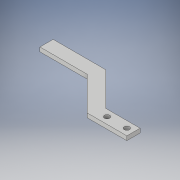
# Autodesk Inventor part: Pinza_dedo
Saved by Autodesk Inventor 2019 (Build 230136000, 136)
## iProperties
Created: 2020-02-07
Part Number: Pinza_dedo
Material: Generic
Document SubType Name: Modeling
Designer: Omar
Density: 1 g/cm^3
Appearance: Default
Author: Omar
Autodesk Inventor part; units mm, degrees
ref_plane "YZ Plane" through (0, 0, 0) normal (1, 0, 0) x (0, 1, 0)
ref_plane "XZ Plane" through (0, 0, 0) normal (0, 1, 0) x (-1, 0, 0)
ref_plane "XY Plane" through (0, 0, 0) normal (0, 0, 1) x (1, 0, 0)
sketch "Sketch1" plane through (0, 0, 0) normal (0, 1, 0) x (-1, 0, 0)
  line L0 (0, 0) -> (40, 0)
  line L1 (40, 0) -> (40, -10)
  line L2 (40, -10) -> (0, -10)
  line L3 (0, -10) -> (0, 0)
  line L4 (0, -10) -> (7.0711, -2.9289)
  line L5 (7.0711, -2.9289) -> (-21.2132, 25.3553)
  line L6 (-21.2132, 25.3553) -> (-28.2843, 18.2843)
  line L7 (-28.2843, 18.2843) -> (0, -10)
  line L8 (-21.2132, 25.3553) -> (-21.2132, 15.3553)
  line L9 (-21.2132, 15.3553) -> (-51.2132, 15.3553)
  line L10 (-51.2132, 15.3553) -> (-51.2132, 25.3553)
  line L11 (-51.2132, 25.3553) -> (-21.2132, 25.3553)
  circle A0 centre (-31.2132, 20.3553) radius 2
  circle A1 centre (-46.2132, 20.3553) radius 2
  dimension "d0" = 10
  dimension "d1" = 40
  dimension "d2" = 135
  dimension "d3" = 40
  dimension "d4" = 10
  dimension "d14" = 45
  dimension "d15" = 10
  dimension "d16" = 30
  dimension "d17" = 4
  dimension "d18" = 10
  dimension "d19" = 5
  dimension "d22" = 4
  dimension "d23" = 5
  dimension "d24" = 5
  constraints: 24 end point, 6 parallel, 3 perpendicular, 2 centre point, 1 horizontal
  measures "d0" distance of L0.end L1.end
  measures "d1" distance of L1.end L2.end
  measures "d2" angle of L5 L0
  measures "d3" distance between parallel lines of L4 L6
  measures "d4" distance between parallel lines of L7 L5
  measures "d14" angle of L5 L8
  measures "d15" distance of L5.end L8.end
  measures "d16" distance of L10.end L5.end
  measures "d17" diameter of A0
  measures "d18" distance from line of L8 A0.centre
  measures "d19" distance from line of L11 A0.centre
  measures "d22" diameter of A1
  measures "d23" distance from line of L9 A1.centre
  measures "d24" distance from line of L10 A1.centre
extrude "Extrusion4" add sketch "Sketch1" along normal blind 3.18
body "Solid4"
